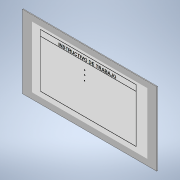
# Autodesk Inventor part: Tabla_Instructivo
Saved by Autodesk Inventor 2021 (Build 250183000, 183)
## iProperties
Created: 2021-07-11
Part Number: Tabla_Instructivo
Material: Generic
Document SubType Name: Modeling
Designer: Nelson
Density: 1 g/cm^3
Appearance: Default
Author: Nelson
Autodesk Inventor part; units mm, degrees
ref_plane "YZ Plane" through (0, 0, 0) normal (1, 0, 0) x (0, 1, 0)
ref_plane "XZ Plane" through (0, 0, 0) normal (0, 1, 0) x (-1, 0, 0)
ref_plane "XY Plane" through (0, 0, 0) normal (0, 0, 1) x (1, 0, 0)
sketch "Sketch1" plane through (0, 0, 0) normal (0, 0, 1) x (1, 0, 0)
  line L0 (0, 0) -> (550, 0)
  line L1 (550, 0) -> (550, 300)
  line L2 (550, 300) -> (0, 300)
  line L3 (0, 300) -> (0, 0)
  dimension "d0" = 300
  dimension "d1" = 550
  constraints: 8 end point, 2 parallel, 1 horizontal, 1 perpendicular
  measures "d0" distance of L0.end L1.end
  measures "d1" distance of L1.end L2.end
extrude "Extrusion1" add sketch "Sketch1" along normal blind 3
sketch "Sketch3" plane through (0, 0, 3) normal (0, 0, 1) x (1, 0, 0)
  line L0 (38, 275.818) -> (512, 275.818) construction
  line L1 (512, 275.818) -> (512, 24.1834) construction
  line L2 (512, 24.1834) -> (38, 24.1834) construction
  line L3 (38, 24.1834) -> (38, 275.818) construction
  line L4 (0, 300) -> (0, 0) projected
  line L5 (550, 0) -> (550, 300) projected
  line L6 (550, 300) -> (0, 300) projected
  line L7 (0, 0) -> (550, 0) projected
  dimension "d37" = 38
  dimension "d38" = 38
  dimension "d39" = 24.182
  dimension "d40" = 24.1834
  constraints: 2 other
  measures "d37" distance between parallel lines of L3 L4
  measures "d38" distance between parallel lines of L5 L1
  measures "d39" distance between parallel lines of L6 L0
  measures "d40" distance between parallel lines of L7 L2
decal "Decal2"
body "Solid1"
